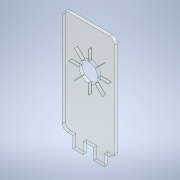
# Autodesk Inventor part: Scheibe
Saved by Autodesk Inventor 2021 (Build 250183000, 183)
## iProperties
Created: 2021-03-05
Part Number: Scheibe
Material: Glas
Document SubType Name: Modeling
Designer: Tilman
Density: 2.18 g/cm^3
Appearance: Klar
Author: Tilman
Autodesk Inventor part; units mm, degrees
ref_plane "YZ Plane" through (0, 0, 0) normal (1, 0, 0) x (0, 1, 0)
ref_plane "XZ Plane" through (0, 0, 0) normal (0, 1, 0) x (-1, 0, 0)
ref_plane "XY Plane" through (0, 0, 0) normal (0, 0, 1) x (1, 0, 0)
sketch "Skizze1" plane through (0, 0, 0) normal (0, 0, 1) x (1, 0, 0)
  line L0 (0, 5) -> (0, 95)
  line L1 (5, 100) -> (45, 100)
  line L2 (50, 95) -> (50, 5)
  arc A0 (5, 100) -> (0, 95) centre (5, 95) ccw
  arc A1 (50, 95) -> (45, 100) centre (45, 95) ccw
  arc A2 (45, 0) -> (50, 5) centre (45, 5) ccw
  arc A3 (0, 5) -> (5, 0) centre (5, 5) ccw
  line L3 (10, 0) -> (10, -11)
  line L4 (10, -11) -> (20, -11)
  line L5 (20, -11) -> (20, 0)
  line L6 (30, 0) -> (30, -11)
  line L7 (30, -11) -> (40, -11)
  line L8 (40, -11) -> (40, 0)
  line L9 (5, 0) -> (10, 0)
  line L10 (20, 0) -> (30, 0)
  line L11 (40, 0) -> (45, 0)
  circle A4 centre (25, 60) radius 9
  line L12 (24.75, 68.9965) -> (24.75, 78.9965)
  line L13 (24.75, 78.9965) -> (25.25, 78.9965)
  line L14 (25.25, 78.9965) -> (25.25, 68.9965)
  line L15 (18.4617, 66.1847) -> (11.3907, 73.2558)
  line L16 (11.3907, 73.2558) -> (11.7442, 73.6093)
  line L17 (11.7442, 73.6093) -> (18.8153, 66.5383)
  line L18 (16.0035, 59.75) -> (6.0035, 59.75)
  line L19 (6.0035, 59.75) -> (6.0035, 60.25)
  line L20 (6.0035, 60.25) -> (16.0035, 60.25)
  line L21 (18.8153, 53.4617) -> (11.7442, 46.3907)
  line L22 (11.7442, 46.3907) -> (11.3907, 46.7442)
  line L23 (11.3907, 46.7442) -> (18.4617, 53.8153)
  line L24 (25.25, 51.0035) -> (25.25, 41.0035)
  line L25 (25.25, 41.0035) -> (24.75, 41.0035)
  line L26 (24.75, 41.0035) -> (24.75, 51.0035)
  line L27 (31.5383, 53.8153) -> (38.6093, 46.7442)
  line L28 (38.6093, 46.7442) -> (38.2558, 46.3907)
  line L29 (38.2558, 46.3907) -> (31.1847, 53.4617)
  line L30 (33.9965, 60.25) -> (43.9965, 60.25)
  line L31 (43.9965, 60.25) -> (43.9965, 59.75)
  line L32 (43.9965, 59.75) -> (33.9965, 59.75)
  line L33 (31.1847, 66.5383) -> (38.2558, 73.6093)
  line L34 (38.2558, 73.6093) -> (38.6093, 73.2558)
  line L35 (38.6093, 73.2558) -> (31.5383, 66.1847)
  point P0 (0, 0)
  point P1 (25, 0)
  point P2 (31.1847, 66.5383)
  point P3 (33.9965, 59.75)
  point P4 (31.5383, 53.8153)
  point P5 (31.1847, 53.4617)
  point P6 (25.25, 51.0035)
  point P7 (24.75, 51.0035)
  point P8 (18.8153, 53.4617)
  point P9 (18.4617, 53.8153)
  point P10 (16.0035, 59.75)
  point P11 (16.0035, 60.25)
  point P12 (18.4617, 66.1847)
  point P13 (18.8153, 66.5383)
  dimension "d1" = 50
  dimension "d3" = 5
  dimension "d4" = 11
  dimension "d5" = 10
  dimension "d6" = 100
  dimension "d9" = 60
  dimension "d10" = 18
  dimension "d11" = 0.5
  dimension "d12" = 10
  dimension "d15" = 360
  constraints: 72 end point, 10 point on circle, 7 tangent, 6 equal length, 5 centre point, 5 vertical, 4 horizontal, 3 equal radius, 3 horizontal alignment, 2 collinear, 2 parallel, 2 perpendicular, 2 vertical alignment, 1 midpoint, 57 other
  measures "d1" distance between parallel lines of L2 L0
  measures "d3" radius of A0
  measures "d4" distance of L3.start L3.end
  measures "d5" distance of L3.end L4.end
  measures "d6" distance between parallel lines of L10 L1
  measures "d9" distance from line of L10 A4.centre
  measures "d10" diameter of A4
  measures "d11" distance of L12.end L13.end
  measures "d12" distance of L13.end L14.end
extrude "Extrusion1" add sketch "Skizze1" along normal blind 3
